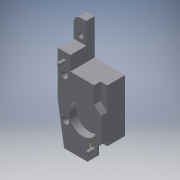
# Autodesk Inventor part: J024 mount
Saved by Autodesk Inventor 2016 SP1 (Build 200210100, 210)
## iProperties
Created: 2016-09-17
Part Number: J024 mount
Material: Generic
Document SubType Name: Modeling
Designer: benja
Density: 1 g/cm^3
Appearance: Default
Author: benja
Autodesk Inventor part; units mm, degrees
ref_plane "YZ Plane" through (0, 0, 0) normal (1, 0, 0) x (0, 1, 0)
ref_plane "XZ Plane" through (0, 0, 0) normal (0, 1, 0) x (-1, 0, 0)
ref_plane "XY Plane" through (0, 0, 0) normal (0, 0, 1) x (1, 0, 0)
sketch "Sketch1" plane through (0, 0, 0) normal (0, 0, 1) x (1, 0, 0)
  line L0 (0, 0) -> (0, -14.67)
  line L1 (0, -14.67) -> (-11, -14.67)
  line L2 (-11, -14.67) -> (-11.7, -8.67)
  line L3 (-11.7, -8.67) -> (-11.7, 9.98)
  line L4 (-11.7, 9.98) -> (-8.4, 9.98)
  line L5 (-8.4, 9.98) -> (-8.4, 0)
  line L6 (-8.4, 0) -> (0, 0)
  dimension "d0" = 24.65
  dimension "d1" = 6
  dimension "d2" = 11.7
  dimension "d3" = 8.4
  dimension "d4" = 14.67
  dimension "d5" = 11
  constraints: 14 end point, 4 perpendicular, 1 parallel, 1 vertical
  measures "d0" distance between parallel lines of L1 L4
  measures "d1" distance from line of L1 L2.end
  measures "d2" distance between parallel lines of L0 L3
  measures "d3" distance between parallel lines of L0 L5
  measures "d4" distance between parallel lines of L1 L6
  measures "d5" distance of L0.end L1.end
extrude "Extrusion1" add sketch "Sketch1" along normal blind 6.75
sketch "Sketch2" plane through (0, 0, 6.75) normal (0, 0, 1) x (1, 0, 0)
  line L0 (0, -14.67) -> (0, 0) projected
  line L1 (0, 0) -> (-8.4, 0) projected
  line L2 (-8.4, 0) -> (-8.4, 9.98) projected
  line L3 (-8.4, 9.98) -> (-11.7, 9.98) projected
  line L4 (-11.7, 9.98) -> (-11.7, -8.67) projected
  line L5 (-11.7, -8.67) -> (-11, -14.67) projected
  line L6 (-11, -14.67) -> (0, -14.67) projected
  line L7 (-11.7, 9.98) -> (-8.4, 9.98)
  line L8 (-8.4, 9.98) -> (-8.4, 3.98)
  line L9 (-8.4, 3.98) -> (-11.7, 3.98)
  line L10 (-11.7, 3.98) -> (-11.7, 9.98)
  dimension "d8" = 6
  constraints: 8 end point, 2 parallel, 1 horizontal, 1 perpendicular, 1 point on line
  measures "d8" distance between parallel lines of L3 L9
extrude "Extrusion2" cut sketch "Sketch2" against normal blind 4.42 contours L9 L4 L3 L2
fillet "Fillet1" radius 2 1 edges at (-11.7, 9.98, 1.165)
sketch "Sketch3" plane through (0, 0, 6.75) normal (0, 0, 1) x (1, 0, 0)
  line L0 (-11.7, 3.98) -> (-11.7, -8.67) projected
  line L1 (-11, -14.67) -> (0, -14.67) projected
  line L2 (-8.4, 3.98) -> (-11.7, 3.98) projected
  point P0 (0, 0)
  point P1 (-9.79, -12.45)
  point P2 (-9.8, -1.62)
  point P3 (-9.8, 5.76)
  dimension "d13" = 1.9
  dimension "d14" = 1.9
  dimension "d15" = 2.22
  dimension "d26" = 5.6
  dimension "d27" = 1.78
  dimension "d28" = 1.21
  measures "d13" distance from line of L0 point (-9.8, -1.62)
  measures "d14" distance from line of L0 point (-9.8, 5.76)
  measures "d15" distance from line of L1 point (-9.79, -12.45)
  measures "d26" distance from line of L2 point (-9.8, -1.62)
  measures "d27" distance from line of point (-9.8, 5.76) L2
  measures "d28" horizontal distance of L1.start point (-9.79, -12.45)
hole "Hole1" at (-9.79, -12.45, 6.75) at (-9.8, -1.62, 6.75) at (-9.8, 5.76, 6.75) direction (0, 0, -1) diameter 1.45 end through all
sketch "Sketch4" plane through (0, 0, 6.75) normal (0, 0, 1) x (1, 0, 0)
  line L0 (0, -14.67) -> (0, 0) projected
  line L1 (0, -6.52) -> (-1.87, -4.65)
  line L2 (-1.87, -4.65) -> (-1.87, 0)
  line L3 (0, 0) -> (-8.4, 0) projected
  line L4 (0, -13.46) -> (-1.21, -14.67)
  line L5 (-11, -14.67) -> (0, -14.67) projected
  dimension "d29" = 1.87
  dimension "d30" = 135
  dimension "d31" = 1.21
  dimension "d32" = 1.21
  dimension "d34" = 4.65
  constraints: 6 end point, 4 point on line, 1 vertical
  measures "d29" distance between parallel lines of L0 L2
  measures "d30" angle of L2 L1
  measures "d31" distance of L0.start L4.start
  measures "d32" distance of L0.start L4.end
  measures "d34" distance from line of L3 L1.end
extrude "Extrusion3" cut sketch "Sketch4" against normal blind 1.8
sketch "Sketch5" plane through (0, 0, 6.75) normal (0, 0, 1) x (1, 0, 0)
  line L0 (-11, -14.67) -> (-1.21, -14.67) projected
  line L1 (-1.21, -14.67) -> (-1.21, -16.67)
  line L2 (-1.21, -16.67) -> (-3.21, -18.67)
  line L3 (-3.21, -18.67) -> (-10.5333, -18.67)
  line L4 (-11.7, -8.67) -> (-11, -14.67) projected
  line L5 (-10.5333, -18.67) -> (-11, -14.67)
  point P0 (0, 0)
  dimension "d37" = 4
  dimension "d38" = 135
  dimension "d39" = 2
  constraints: 8 end point, 1 collinear, 1 perpendicular, 1 vertical
  measures "d37" distance between parallel lines of L0 L3
  measures "d38" angle of L1 L2
  measures "d39" distance from line of L3 L1.end
extrude "Extrusion4" add sketch "Sketch5" against normal blind 0.7
ref_plane "Work Plane1" through (-2.91, -16.67, 6.75) normal (1, 0, 0) x (0, 0, -1)
sketch "Sketch6" plane through (-2.91, -16.67, 6.75) normal (1, 0, 0) x (0, 0, -1)
  line L0 (0.7, 2) -> (0.7, -0.6)
  line L1 (0.7, 2) -> (0.7, 0)
  line L2 (0.7, 2) -> (4.5, 2)
  line L3 (4.5, 2) -> (0.7, -0.6)
  line L4 (0.7, 2) -> (0.7, 0) projected
  line L5 (6.75, 2) -> (1.8, 2) projected
  point P0 (6.75, 16.87)
  dimension "d42" = 3.8
  dimension "d43" = 2.6
  constraints: 8 end point, 2 collinear, 1 point on line
  measures "d42" distance of L0.start L2.end
  measures "d43" distance from line of L2 L0.end
extrude "Extrusion5" add sketch "Sketch6" against normal blind 0.7
pattern_linear "Rectangular Pattern1" count 3 spacing 3 along (-1, 0, 0) of "Extrusion5"
sketch "Sketch7" plane through (0, 0, 6.75) normal (0, 0, 1) x (1, 0, 0)
  circle A0 centre (-2.8, -15.87) radius 0.5
  circle A1 centre (-9.95, 1.68) radius 0.5
  line L0 (-11.7, 3.98) -> (-11.7, -8.67) projected
  line L1 (-8.4, 3.98) -> (-11.7, 3.98) projected
  line L2 (-1.21, -14.67) -> (-1.21, -16.67) projected
  line L3 (0, -14.67) -> (-1.21, -14.67) projected
  line L4 (-3.21, -18.67) -> (-10.5333, -18.67) projected
  line L5 (0, -13.46) -> (0, -6.52) projected
  point P0 (0, 0)
  dimension "d50" = 1
  dimension "d51" = 1
  dimension "d85" = 1.25
  dimension "d86" = 1.8
  dimension "d87" = 2.3
  dimension "d88" = 2.3
  constraints: 2 centre point
  measures "d50" diameter of A0
  measures "d51" diameter of A1
  measures "d85" distance edge to line of A1 L0
  measures "d86" distance edge to line of A1 L1
  measures "d87" distance edge to line of A0 L4
  measures "d88" distance edge to line of A0 L5
extrude "Extrusion6" add sketch "Sketch7" along normal blind 1.05
fillet "Fillet2" radius 0.2 2 edges at (-3.3, -15.87, 7.8) (-10.45, 1.68, 7.8)
sketch "Sketch8" plane through (0, 0, 6.75) normal (0, 0, 1) x (1, 0, 0)
  circle A0 centre (-4.4, -10.37) radius 3.9
  line L0 (0, -13.46) -> (0, -6.52) projected
  line L1 (-3.21, -18.67) -> (-10.5333, -18.67) projected
  point P0 (0, 0)
  dimension "d59" = 7.8
  dimension "d60" = 0.5
  dimension "d61" = 4.4
  constraints: 1 centre point
  measures "d59" diameter of A0
  measures "d60" distance edge to line of A0 L0
  measures "d61" distance edge to line of A0 L1
extrude "Extrusion7" cut sketch "Sketch8" against normal blind 2
chamfer "Chamfer1" distance 0.2 angle 45 5 edges at (-9.8, 6.485, 0) (-9.8, -0.895, 0) (-9.79, -11.725, 0) (-9.79, -11.725, 6.75) (-9.8, -0.895, 6.75)
sketch "Sketch9" plane through (0, 0, 0) normal (0, 0, -1) x (-1, 0, 0)
  circle A0 centre (3.75, -2.92) radius 0.75
  circle A1 centre (8.09, -8.92) radius 0.75
  line L0 (0, 0) -> (0, -14.67) projected
  line L1 (0, -14.67) -> (11, -14.67) projected
  line L2 (11.7, -8.67) -> (11.7, 7.98) projected
  dimension "d67" = 1.5
  dimension "d68" = 1.5
  dimension "d69" = 3
  dimension "d70" = 11
  dimension "d71" = 5
  dimension "d72" = 2.86
  constraints: 2 centre point
  measures "d67" diameter of A0
  measures "d68" diameter of A1
  measures "d69" distance edge to line of A0 L0
  measures "d70" distance edge to line of A0 L1
  measures "d71" distance edge to line of A1 L1
  measures "d72" distance edge to line of A1 L2
extrude "Extrusion8" add sketch "Sketch9" along normal blind 1
chamfer "Chamfer2" distance 0.2 angle 45 2 edges at (-7.34, -8.92, -1) (-3, -2.92, -1)
sketch "Sketch10" plane through (-8.4, 9.98, 2.33) normal (0, 1, 0) x (1, 0, 0)
  line L0 (-1.3, 0) -> (-1.3, 2.33) projected
  line L1 (-1.3, 0) -> (0, 0) projected
  line L2 (0, 2.33) -> (0, 0) projected
  line L3 (-1.3, 2.33) -> (0, 2.33) projected
  line L4 (-1.3, 0) -> (-0.3, 0)
  line L5 (-0.3, 0) -> (-0.3, 1)
  line L6 (-0.3, 1) -> (-1.3, 1)
  line L7 (-1.3, 1) -> (-1.3, 0)
  point P0 (8.4, 2.33)
  dimension "d78" = 1
  dimension "d79" = 1
  constraints: 8 end point, 2 parallel, 1 horizontal, 1 perpendicular
  measures "d78" distance of L6.end L5.end
  measures "d79" distance of L5.end L4.end
extrude "Extrusion9" add sketch "Sketch10" along normal blind 1.78 contours L0 L6 L5 L1
sketch "Sketch11" plane through (0, 0, 6.75) normal (0, 0, 1) x (1, 0, 0)
  arc A0 (-6.9282, -7.4005) -> (-8.036, -8.9596) centre (-8.2, -7.67) ccw
  circle A1 centre (-4.4, -10.37) radius 3.9 projected
  line L0 (-3.21, -18.67) -> (-10.5333, -18.67) projected
  line L1 (-11.7, 3.98) -> (-11.7, -8.67) projected
  point P0 (0, 0)
  dimension "d82" = 9.7
  dimension "d83" = 2.2
  dimension "d84" = 2.6
  constraints: 4 point on circle, 1 centre point
  measures "d82" distance edge to line of A0 L0
  measures "d83" distance edge to line of A0 L1
  measures "d84" diameter of A0
extrude "Extrusion10" add sketch "Sketch11" along normal blind 0.25 contours A1 A0
equation "\"d14\" = d13"
equation "\"d32\" = d31"
equation "\"d68\" = d67"
body "Solid1"
